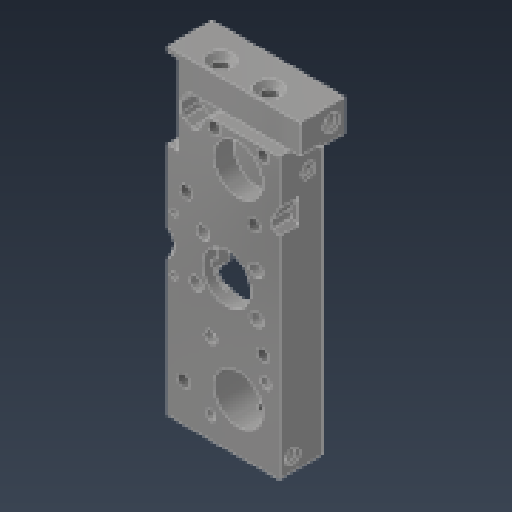
# Autodesk Inventor part: LeftGearbox
Saved by Autodesk Inventor 2027.1 (Build 311270010, 270A)
## iProperties
Created: 2026-04-13
Part Number: LeftGearbox
Material: Steel
Document SubType Name: Modeling
Designer: szymo
Density: 7.85 g/cm^3
Appearance: Nylon 6(1)
Mass: 68.9127 g
Surface Area: 68.8445 cm^2
Volume: 8.77869 cm^3
Author: szymo
Autodesk Inventor part; units mm, degrees
(part 1 of 2)
ref_plane "YZ Plane" through (0, 0, 0) normal (1, 0, 0) x (0, 1, 0)
ref_plane "XZ Plane" through (0, 0, 0) normal (0, 1, 0) x (-1, 0, 0)
ref_plane "XY Plane" through (0, 0, 0) normal (0, 0, 1) x (1, 0, 0)
sketch "Sketch1" plane through (0, 0, 0) normal (0, 0, 1) x (1, 0, 0)
  circle A0 centre (14.7, -55.637072) radius 14.7 construction
  circle A1 centre (14.7, -55.637072) radius 14 construction
  circle A2 centre (14.7, -55.637072) radius 5
  circle A3 centre (14.7, -14.7) radius 5
  circle A4 centre (14.7, -14.7) radius 14 construction
  circle A5 centre (14.7, -14.7) radius 14.7 construction
  circle A6 centre (12.35, -35.272213) radius 5
  circle A7 centre (9.001972, -47.419258) radius 8 construction
  circle A8 centre (9.001972, -47.419258) radius 4.2 construction
  circle A9 centre (12.35, -35.272213) radius 9.6 construction
  line L0 (23.1, -65.837072) -> (0, -65.837072)
  line L1 (0, -65.837072) -> (0, 0)
  line L2 (0, 0) -> (23.1, 0)
  line L3 (23.1, 0) -> (23.1, -65.837072)
  circle A10 centre (12.35, -35.272213) radius 10
  circle A11 centre (9.001972, -47.419258) radius 8.4
  line L4 (29.4, -55.637072) -> (23.1, -55.637072)
  line L5 (14.7, -55.637072) -> (23.1, -55.637072) construction
  line L6 (5.96251, -12.542159) -> (1.960875, -10.231814) construction
  arc A12 (4.460875, -5.901687) -> (1.960875, -10.231814) centre (14.7, -14.7) ccw construction
  line L7 (4.460875, -5.901687) -> (8.46251, -8.212032)
  arc A13 (8.46251, -8.212032) -> (5.96251, -12.542159) centre (14.7, -14.7) ccw construction
  arc A14 (24.939125, -23.498313) -> (27.439125, -19.168186) centre (14.7, -14.7) ccw
  line L8 (27.439125, -19.168186) -> (23.43749, -16.857841)
  arc A15 (20.93749, -21.187968) -> (23.43749, -16.857841) centre (14.7, -14.7) ccw construction
  line L9 (20.93749, -21.187968) -> (24.939125, -23.498313) construction
  line L10 (20.93749, -21.187968) -> (23.43749, -16.857841)
  line L11 (4.460875, -5.901687) -> (23.1, -5.901687)
  line L12 (5.96251, -12.542159) -> (23.1, -12.542159)
  line L13 (5.96251, -12.542159) -> (8.46251, -8.212032)
  line L14 (23.1, -6.5) -> (27.4, -6.5)
  line L15 (27.4, -6.5) -> (27.4, 0)
  line L16 (27.4, 0) -> (23.1, 0)
  circle A16 centre (9.001972, -47.419258) radius 4.6
  circle A17 centre (14.7, -55.637072) radius 14.7
  circle A18 centre (14.7, -55.637072) radius 14
  circle A19 centre (9.043146, -61.293926) radius 1.05643
  circle A20 centre (20.356854, -49.980218) radius 1.05643
  circle A21 centre (14.7, -55.637072) radius 5
  circle A22 centre (14.7, -55.637072) radius 14
  circle A23 centre (14.7, -14.7) radius 14.7
  circle A24 centre (14.7, -14.7) radius 14
  line L17 (6.887728, -8.457532) -> (4.702907, -7.196125)
  arc A25 (4.702907, -7.196125) -> (3.202907, -9.794201) centre (14.7, -14.7) ccw
  line L18 (3.202907, -9.794201) -> (5.387728, -11.055608)
  arc A26 (6.887728, -8.457532) -> (5.387728, -11.055608) centre (14.7, -14.7) ccw
  arc A27 (24.697093, -22.203875) -> (26.197093, -19.605799) centre (14.7, -14.7) ccw
  line L19 (26.197093, -19.605799) -> (24.012272, -18.344392)
  arc A28 (22.512272, -20.942468) -> (24.012272, -18.344392) centre (14.7, -14.7) ccw
  line L20 (22.512272, -20.942468) -> (24.697093, -22.203875)
  circle A29 centre (14.7, -14.7) radius 5
  circle A30 centre (14.7, -14.7) radius 14
  arc A31 (9.833797, -26.007834) -> (9.773924, -27.434717) centre (15.759046, -26.971155) ccw
  arc A32 (10.322105, -25.888842) -> (9.833797, -26.007834) centre (12.35, -35.272213) ccw
  arc A33 (11.031695, -27.128223) -> (10.322105, -25.888842) centre (5.50427, -29.470047) ccw
  arc A34 (11.459725, -27.070389) -> (11.031695, -27.128223) centre (12.35, -35.272213) ccw
  arc A35 (11.814954, -25.687134) -> (11.459725, -27.070389) centre (17.410437, -27.861334) ccw
  arc A36 (12.317332, -25.672268) -> (11.814954, -25.687134) centre (12.35, -35.272213) ccw
  arc A37 (12.753733, -27.032097) -> (12.317332, -25.672268) centre (6.860203, -28.173531) ccw
  arc A38 (13.184434, -27.06452) -> (12.753733, -27.032097) centre (12.35, -35.272213) ccw
  arc A39 (13.819496, -25.785349) -> (13.184434, -27.06452) centre (18.840663, -29.075403) ccw
  arc A40 (14.313986, -25.875258) -> (13.819496, -25.785349) centre (12.35, -35.272213) ccw
  arc A41 (14.458127, -27.296105) -> (14.313986, -25.875258) centre (8.456067, -27.187262) ccw
  arc A42 (14.872675, -27.417366) -> (14.458127, -27.296105) centre (12.35, -35.272213) ccw
  arc A43 (15.759814, -26.298185) -> (14.872675, -27.417366) centre (19.987215, -30.560303) ccw
  arc A44 (16.224805, -26.48894) -> (15.759814, -26.298185) centre (12.35, -35.272213) ccw
  arc A45 (16.070386, -27.908706) -> (16.224805, -26.48894) centre (10.222115, -26.554343) ccw
  arc A46 (16.450663, -28.113507) -> (16.070386, -27.908706) centre (12.35, -35.272213) ccw
  arc A47 (17.551107, -27.20323) -> (16.450663, -28.113507) centre (20.799985, -32.251136) ccw
  arc A48 (17.966277, -27.486493) -> (17.551107, -27.20323) centre (12.35, -35.272213) ccw
  arc A49 (17.520045, -28.843128) -> (17.966277, -27.486493) centre (12.081161, -26.302437) ccw
  arc A50 (17.849432, -29.122518) -> (17.520045, -28.843128) centre (12.35, -35.272213) ccw
  arc A51 (19.115086, -28.460927) -> (17.849432, -29.122518) centre (21.24345, -34.074005) ccw
  arc A52 (19.46229, -28.824319) -> (19.115086, -28.460927) centre (12.35, -35.272213) ccw
  arc A53 (18.743749, -30.058532) -> (19.46229, -28.824319) centre (13.951957, -26.442554) ccw
  arc A54 (19.00785, -30.4003) -> (18.743749, -30.058532) centre (12.35, -35.272213) ccw
  arc A55 (20.383398, -30.01631) -> (19.00785, -30.4003) centre (21.298228, -35.94924) ccw
  arc A56 (20.647462, -30.443949) -> (20.383398, -30.01631) centre (12.35, -35.272213) ccw
  arc A57 (19.688016, -31.501799) -> (20.647462, -30.443949) centre (15.75274, -26.968568) ccw
  arc A58 (19.875288, -31.891008) -> (19.688016, -31.501799) centre (12.35, -35.272213) ccw
  arc A59 (21.300613, -31.801402) -> (19.875288, -31.891008) centre (20.961926, -37.794887) ccw
  arc A60 (21.469995, -32.274598) -> (21.300613, -31.801402) centre (12.35, -35.272213) ccw
  arc A61 (20.311576, -33.10985) -> (21.469995, -32.274598) centre (17.404807, -27.857492) ccw
  arc A62 (20.413834, -33.529491) -> (20.311576, -33.10985) centre (12.35, -35.272213) ccw
  arc A63 (21.826643, -33.738185) -> (20.413834, -33.529491) centre (20.249241, -39.53028) ccw
  arc A64 (21.89394, -34.236256) -> (21.826643, -33.738185) centre (12.35, -35.272213) ccw
  arc A65 (20.587177, -34.812408) -> (21.89394, -34.236256) centre (18.835954, -29.070475) ccw
  arc A66 (20.599952, -35.244139) -> (20.587177, -34.812408) centre (12.35, -35.272213) ccw
  arc A67 (21.938498, -35.742012) -> (20.599952, -35.244139) centre (19.191321, -41.079576) ccw
  arc A68 (21.90077, -36.243191) -> (21.938498, -35.742012) centre (12.35, -35.272213) ccw
  arc A69 (20.502773, -36.535061) -> (21.90077, -36.243191) centre (19.983634, -30.554504) ccw
  arc A70 (20.425508, -36.960014) -> (20.502773, -36.535061) centre (12.35, -35.272213) ccw
  arc A71 (21.631289, -37.725306) -> (20.425508, -36.960014) centre (17.834403, -42.375062) ccw
  arc A72 (21.490185, -38.207689) -> (21.631289, -37.725306) centre (12.35, -35.272213) ccw
  arc A73 (20.062055, -38.202522) -> (21.490185, -38.207689) centre (20.797688, -32.244719) ccw
  arc A74 (19.898125, -38.602124) -> (20.062055, -38.202522) centre (12.35, -35.272213) ccw
  arc A75 (20.918444, -39.601389) -> (19.898125, -38.602124) centre (16.237791, -43.360119) ccw
  arc A76 (20.68013, -40.043893) -> (20.918444, -39.601389) centre (12.35, -35.272213) ccw
  arc A77 (19.284282, -39.741914) -> (20.68013, -40.043893) centre (21.242537, -34.06725) ccw
  arc A78 (19.040853, -40.0987) -> (19.284282, -39.741914) centre (12.35, -35.272213) ccw
  arc A79 (19.831117, -41.288266) -> (19.040853, -40.0987) centre (14.471263, -43.991696) ccw
  arc A80 (19.506008, -41.671552) -> (19.831117, -41.288266) centre (12.35, -35.272213) ccw
  arc A81 (18.203449, -41.085958) -> (19.506008, -41.671552) centre (21.298739, -35.942444) ccw
  arc A82 (17.891159, -41.384337) -> (18.203449, -41.085958) centre (12.35, -35.272213) ccw
  arc A83 (18.416829, -42.712212) -> (17.891159, -41.384337) centre (12.612026, -44.24219) ccw
  arc A84 (18.019135, -43.019529) -> (18.416829, -42.712212) centre (12.35, -35.272213) ccw
  arc A85 (16.866791, -42.175915) -> (18.019135, -43.019529) centre (20.963839, -37.788345) ccw
  arc A86 (16.499289, -42.402844) -> (16.866791, -42.175915) centre (12.35, -35.272213) ccw
  arc A87 (16.737391, -43.810995) -> (16.499289, -42.402844) centre (10.741337, -44.100653) ccw
  arc A88 (16.284493, -44.028911) -> (16.737391, -43.810995) centre (12.35, -35.272213) ccw
  arc A89 (15.332728, -42.964146) -> (16.284493, -44.028911) centre (20.252473, -39.524279) ccw
  arc A90 (14.926076, -43.109708) -> (15.332728, -42.964146) centre (12.35, -35.272213) ccw
  arc A91 (14.866203, -44.536592) -> (14.926076, -43.109708) centre (8.940954, -43.57327) ccw
  arc A92 (14.377895, -44.655583) -> (14.866203, -44.536592) centre (12.35, -35.272213) ccw
  arc A93 (13.668305, -43.416203) -> (14.377895, -44.655583) centre (19.19573, -41.074378) ccw
  arc A94 (13.240275, -43.474036) -> (13.668305, -43.416203) centre (12.35, -35.272213) ccw
  arc A95 (12.885046, -44.857291) -> (13.240275, -43.474036) centre (7.289563, -42.683091) ccw
  arc A96 (12.382668, -44.872157) -> (12.885046, -44.857291) centre (12.35, -35.272213) ccw
  arc A97 (11.946267, -43.512328) -> (12.382668, -44.872157) centre (17.839797, -42.370894) ccw
  arc A98 (11.515566, -43.479905) -> (11.946267, -43.512328) centre (12.35, -35.272213) ccw
  arc A99 (10.880504, -44.759076) -> (11.515566, -43.479905) centre (5.859337, -41.469022) ccw
  arc A100 (10.386014, -44.669167) -> (10.880504, -44.759076) centre (12.35, -35.272213) ccw
  arc A101 (10.241873, -43.248321) -> (10.386014, -44.669167) centre (16.243933, -43.357164) ccw
  arc A102 (9.827325, -43.127059) -> (10.241873, -43.248321) centre (12.35, -35.272213) ccw
  arc A103 (8.940186, -44.24624) -> (9.827325, -43.127059) centre (4.712785, -39.984122) ccw
  arc A104 (8.475195, -44.055486) -> (8.940186, -44.24624) centre (12.35, -35.272213) ccw
  arc A105 (8.629614, -42.635719) -> (8.475195, -44.055486) centre (14.477885, -43.990082) ccw
  arc A106 (8.249337, -42.430918) -> (8.629614, -42.635719) centre (12.35, -35.272213) ccw
  arc A107 (7.148893, -43.341196) -> (8.249337, -42.430918) centre (3.900015, -38.293289) ccw
  arc A108 (6.733723, -43.057933) -> (7.148893, -43.341196) centre (12.35, -35.272213) ccw
  arc A109 (7.179955, -41.701297) -> (6.733723, -43.057933) centre (12.618839, -44.241988) ccw
  arc A110 (6.850568, -41.421907) -> (7.179955, -41.701297) centre (12.35, -35.272213) ccw
  arc A111 (5.584914, -42.083498) -> (6.850568, -41.421907) centre (3.45655, -36.470421) ccw
  arc A112 (5.23771, -41.720106) -> (5.584914, -42.083498) centre (12.35, -35.272213) ccw
  arc A113 (5.956251, -40.485894) -> (5.23771, -41.720106) centre (10.748043, -44.101872) ccw
  arc A114 (5.69215, -40.144125) -> (5.956251, -40.485894) centre (12.35, -35.272213) ccw
  arc A115 (4.316602, -40.528115) -> (5.69215, -40.144125) centre (3.401772, -34.595185) ccw
  arc A116 (4.052538, -40.100476) -> (4.316602, -40.528115) centre (12.35, -35.272213) ccw
  arc A117 (5.011984, -39.042627) -> (4.052538, -40.100476) centre (8.94726, -43.575857) ccw
  arc A118 (4.824712, -38.653418) -> (5.011984, -39.042627) centre (12.35, -35.272213) ccw
  arc A119 (3.399387, -38.743023) -> (4.824712, -38.653418) centre (3.738074, -32.749539) ccw
  arc A120 (3.230005, -38.269828) -> (3.399387, -38.743023) centre (12.35, -35.272213) ccw
  arc A121 (4.388424, -37.434575) -> (3.230005, -38.269828) centre (7.295193, -42.686933) ccw
  arc A122 (4.286166, -37.014935) -> (4.388424, -37.434575) centre (12.35, -35.272213) ccw
  arc A123 (2.873357, -36.806241) -> (4.286166, -37.014935) centre (4.450759, -31.014145) ccw
  arc A124 (2.80606, -36.308169) -> (2.873357, -36.806241) centre (12.35, -35.272213) ccw
  arc A125 (4.112823, -35.732018) -> (2.80606, -36.308169) centre (5.864046, -41.47395) ccw
  arc A126 (4.100048, -35.300287) -> (4.112823, -35.732018) centre (12.35, -35.272213) ccw
  arc A127 (2.761502, -34.802414) -> (4.100048, -35.300287) centre (5.508679, -29.464849) ccw
  arc A128 (2.79923, -34.301234) -> (2.761502, -34.802414) centre (12.35, -35.272213) ccw
  arc A129 (4.197227, -34.009364) -> (2.79923, -34.301234) centre (4.716366, -39.989922) ccw
  arc A130 (4.274492, -33.584412) -> (4.197227, -34.009364) centre (12.35, -35.272213) ccw
  arc A131 (3.068711, -32.819119) -> (4.274492, -33.584412) centre (6.865597, -28.169364) ccw
  arc A132 (3.209815, -32.336736) -> (3.068711, -32.819119) centre (12.35, -35.272213) ccw
  arc A133 (4.637945, -32.341904) -> (3.209815, -32.336736) centre (3.902312, -38.299707) ccw
  arc A134 (4.801875, -31.942302) -> (4.637945, -32.341904) centre (12.35, -35.272213) ccw
  arc A135 (3.781556, -30.943037) -> (4.801875, -31.942302) centre (8.462209, -27.184306) ccw
  arc A136 (4.01987, -30.500532) -> (3.781556, -30.943037) centre (12.35, -35.272213) ccw
  arc A137 (5.415718, -30.802512) -> (4.01987, -30.500532) centre (3.457463, -36.477176) ccw
  arc A138 (5.659147, -30.445725) -> (5.415718, -30.802512) centre (12.35, -35.272213) ccw
  arc A139 (4.868883, -29.25616) -> (5.659147, -30.445725) centre (10.228737, -26.552729) ccw
  arc A140 (5.193992, -28.872873) -> (4.868883, -29.25616) centre (12.35, -35.272213) ccw
  arc A141 (6.496551, -29.458467) -> (5.193992, -28.872873) centre (3.401261, -34.601982) ccw
  arc A142 (6.808841, -29.160089) -> (6.496551, -29.458467) centre (12.35, -35.272213) ccw
  arc A143 (6.283171, -27.832213) -> (6.808841, -29.160089) centre (12.087974, -26.302236) ccw
  arc A144 (6.680865, -27.524896) -> (6.283171, -27.832213) centre (12.35, -35.272213) ccw
  arc A145 (7.833209, -28.368511) -> (6.680865, -27.524896) centre (3.736161, -32.75608) ccw
  arc A146 (8.200711, -28.141582) -> (7.833209, -28.368511) centre (12.35, -35.272213) ccw
  arc A147 (7.962609, -26.733431) -> (8.200711, -28.141582) centre (13.958663, -26.443773) ccw
  arc A148 (8.415507, -26.515514) -> (7.962609, -26.733431) centre (12.35, -35.272213) ccw
  arc A149 (9.367272, -27.58028) -> (8.415507, -26.515514) centre (4.447527, -31.020146) ccw
  arc A150 (9.773924, -27.434717) -> (9.367272, -27.58028) centre (12.35, -35.272213) ccw
  circle A151 centre (9.001972, -47.419258) radius 1.25
  arc A152 (9.305411, -54.287558) -> (9.772861, -55.382029) centre (14.106978, -52.883865) ccw
  arc A153 (8.945536, -54.294026) -> (9.305411, -54.287558) centre (9.001972, -47.419258) ccw
  arc A154 (8.517718, -55.404588) -> (8.945536, -54.294026) centre (4.09663, -53.063781) ccw
  arc A155 (8.100462, -55.368301) -> (8.517718, -55.404588) centre (9.001972, -47.419258) ccw
  arc A156 (7.870781, -54.200558) -> (8.100462, -55.368301) centre (12.859266, -53.825841) ccw
  arc A157 (7.517425, -54.132063) -> (7.870781, -54.200558) centre (9.001972, -47.419258) ccw
  arc A158 (6.868057, -55.129407) -> (7.517425, -54.132063) centre (3.030261, -51.920557) ccw
  arc A159 (6.467463, -55.007161) -> (6.868057, -55.129407) centre (9.001972, -47.419258) ccw
  arc A160 (6.485588, -53.817182) -> (6.467463, -55.007161) centre (11.442971, -54.487818) ccw
  arc A161 (6.154195, -53.676717) -> (6.485588, -53.817182) centre (9.001972, -47.419258) ccw
  arc A162 (5.311658, -54.517256) -> (6.154195, -53.676717) centre (2.224885, -50.580604) ccw
  arc A163 (4.945234, -54.314393) -> (5.311658, -54.517256) centre (9.001972, -47.419258) ccw
  arc A164 (5.210374, -53.154187) -> (4.945234, -54.314393) centre (9.919993, -54.840865) ccw
  arc A165 (4.915427, -52.947891) -> (5.210374, -53.154187) centre (9.001972, -47.419258) ccw
  arc A166 (3.916543, -53.594889) -> (4.915427, -52.947891) centre (1.715699, -49.102486) ccw
  arc A167 (3.600305, -53.320274) -> (3.916543, -53.594889) centre (9.001972, -47.419258) ccw
  arc A168 (4.100871, -52.240548) -> (3.600305, -53.320274) centre (8.356893, -54.869553) ccw
  arc A169 (3.855261, -51.977436) -> (4.100871, -52.240548) centre (9.001972, -47.419258) ccw
  arc A170 (2.743686, -52.402616) -> (3.855261, -51.977436) centre (1.524959, -47.550802) ccw
  arc A171 (2.491454, -52.068253) -> (2.743686, -52.402616) centre (9.001972, -47.419258) ccw
  arc A172 (3.205569, -51.116195) -> (2.491454, -52.068253) centre (6.821986, -54.572627) ccw
  arc A173 (3.02003, -50.807768) -> (3.205569, -51.116195) centre (9.001972, -47.419258) ccw
  arc A174 (1.844346, -50.992547) -> (3.02003, -50.807768) centre (1.661, -45.993369) ccw
  arc A175 (1.667144, -50.613049) -> (1.844346, -50.992547) centre (9.001972, -47.419258) ccw
  arc A176 (2.563598, -49.830268) -> (1.667144, -50.613049) centre (5.382355, -53.963064) ccw
  arc A177 (2.446239, -49.490005) -> (2.563598, -49.830268) centre (9.001972, -47.419258) ccw
  arc A178 (1.257829, -49.426308) -> (2.446239, -49.490005) centre (2.117877, -44.498254) ccw
  arc A179 (1.163401, -49.01826) -> (1.257829, -49.426308) centre (9.001972, -47.419258) ccw
  arc A180 (2.203015, -48.438968) -> (1.163401, -49.01826) centre (4.100919, -53.067505) ccw
  arc A181 (2.158965, -48.081741) -> (2.203015, -48.438968) centre (9.001972, -47.419258) ccw
  arc A182 (1.009768, -47.772351) -> (2.158965, -48.081741) centre (2.875622, -43.130802) ccw
  arc A183 (1.002241, -47.353588) -> (1.009768, -47.772351) centre (9.001972, -47.419258) ccw
  arc A184 (2.139578, -47.003102) -> (1.002241, -47.353588) centre (3.033682, -51.925091) ccw
  arc A185 (2.170763, -46.644523) -> (2.139578, -47.003102) centre (9.001972, -47.419258) ccw
  arc A186 (1.111004, -46.102963) -> (2.170763, -46.644523) centre (3.901117, -41.950775) ccw
  arc A187 (1.190708, -45.691785) -> (1.111004, -46.102963) centre (9.001972, -47.419258) ccw
  arc A188 (2.376062, -45.585425) -> (1.190708, -45.691785) centre (2.227288, -50.585751) ccw
  arc A189 (2.481118, -45.241165) -> (2.376062, -45.585425) centre (9.001972, -47.419258) ccw
  arc A190 (1.557114, -44.491103) -> (2.481118, -45.241165) centre (5.149545, -41.009747) ccw
  arc A191 (1.720565, -44.105482) -> (1.557114, -44.491103) centre (9.001972, -47.419258) ccw
  arc A192 (2.902129, -44.247894) -> (1.720565, -44.105482) centre (1.71698, -49.10802) ccw
  arc A193 (3.076465, -43.932999) -> (2.902129, -44.247894) centre (9.001972, -47.419258) ccw
  arc A194 (2.328599, -43.007217) -> (3.076465, -43.932999) centre (6.566342, -40.348846) ccw
  arc A195 (2.568654, -42.664006) -> (2.328599, -43.007217) centre (9.001972, -47.419258) ccw
  arc A196 (3.694789, -43.048968) -> (2.568654, -42.664006) centre (1.525061, -47.556481) ccw
  arc A197 (3.930785, -42.7772) -> (3.694789, -43.048968) centre (9.001972, -47.419258) ccw
  arc A198 (3.391744, -41.716159) -> (3.930785, -42.7772) centre (8.089587, -39.996955) ccw
  arc A199 (3.697909, -41.430358) -> (3.391744, -41.716159) centre (9.001972, -47.419258) ccw
  arc A200 (4.719398, -42.041044) -> (3.697909, -41.430358) centre (1.659919, -45.998945) ccw
  arc A201 (5.006741, -41.824282) -> (4.719398, -42.041044) centre (9.001972, -47.419258) ccw
  arc A202 (4.700082, -40.674353) -> (5.006741, -41.824282) centre (9.652709, -39.969455) ccw
  arc A203 (5.058978, -40.458453) -> (4.700082, -40.674353) centre (9.001972, -47.419258) ccw
  arc A204 (5.931176, -41.268173) -> (5.058978, -40.458453) centre (2.11566, -44.503484) ccw
  arc A205 (6.257307, -41.11589) -> (5.931176, -41.268173) centre (9.001972, -47.419258) ccw
  arc A206 (6.196433, -39.927332) -> (6.257307, -41.11589) centre (11.18739, -40.267547) ccw
  arc A207 (6.592375, -39.790769) -> (6.196433, -39.927332) centre (9.001972, -47.419258) ccw
  arc A208 (7.277163, -40.764135) -> (6.592375, -39.790769) centre (2.872366, -43.135456) ccw
  arc A209 (7.627829, -40.682986) -> (7.277163, -40.764135) centre (9.001972, -47.419258) ccw
  arc A210 (7.815399, -39.507744) -> (7.627829, -40.682986) centre (12.626557, -40.878203) ccw
  arc A211 (8.231082, -39.456486) -> (7.815399, -39.507744) centre (9.001972, -47.419258) ccw
  arc A212 (8.698532, -40.550958) -> (8.231082, -39.456486) centre (3.896965, -41.954651) ccw
  arc A213 (9.058407, -40.544489) -> (8.698532, -40.550958) centre (9.001972, -47.419258) ccw
  arc A214 (9.486225, -39.433928) -> (9.058407, -40.544489) centre (13.907313, -41.774735) ccw
  arc A215 (9.903481, -39.470215) -> (9.486225, -39.433928) centre (9.001972, -47.419258) ccw
  arc A216 (10.133163, -40.637958) -> (9.903481, -39.470215) centre (5.144678, -41.012675) ccw
  arc A217 (10.486518, -40.706453) -> (10.133163, -40.637958) centre (9.001972, -47.419258) ccw
  arc A218 (11.135886, -39.709108) -> (10.486518, -40.706453) centre (14.973682, -42.917959) ccw
  arc A219 (11.53648, -39.831355) -> (11.135886, -39.709108) centre (9.001972, -47.419258) ccw
  arc A220 (11.518355, -41.021333) -> (11.53648, -39.831355) centre (6.560972, -40.350698) ccw
  arc A221 (11.849748, -41.161799) -> (11.518355, -41.021333) centre (9.001972, -47.419258) ccw
  arc A222 (12.692286, -40.321259) -> (11.849748, -41.161799) centre (15.779059, -44.257911) ccw
  arc A223 (13.058709, -40.524123) -> (12.692286, -40.321259) centre (9.001972, -47.419258) ccw
  arc A224 (12.793569, -41.684329) -> (13.058709, -40.524123) centre (8.08395, -39.997651) ccw
  arc A225 (13.088516, -41.890625) -> (12.793569, -41.684329) centre (9.001972, -47.419258) ccw
  arc A226 (14.0874, -41.243627) -> (13.088516, -41.890625) centre (16.288244, -45.73603) ccw
  arc A227 (14.403638, -41.518241) -> (14.0874, -41.243627) centre (9.001972, -47.419258) ccw
  arc A228 (13.903073, -42.597968) -> (14.403638, -41.518241) centre (9.64705, -39.968963) ccw
  arc A229 (14.148683, -42.861079) -> (13.903073, -42.597968) centre (9.001972, -47.419258) ccw
  arc A230 (15.260257, -42.4359) -> (14.148683, -42.861079) centre (16.478984, -47.287714) ccw
  arc A231 (15.512489, -42.770262) -> (15.260257, -42.4359) centre (9.001972, -47.419258) ccw
  arc A232 (14.798374, -43.722321) -> (15.512489, -42.770262) centre (11.181957, -40.265889) ccw
  arc A233 (14.983913, -44.030748) -> (14.798374, -43.722321) centre (9.001972, -47.419258) ccw
  arc A234 (16.159597, -43.845969) -> (14.983913, -44.030748) centre (16.342943, -48.845147) ccw
  arc A235 (16.336799, -44.225467) -> (16.159597, -43.845969) centre (9.001972, -47.419258) ccw
  arc A236 (15.440345, -45.008248) -> (16.336799, -44.225467) centre (12.621588, -40.875452) ccw
  arc A237 (15.557704, -45.348511) -> (15.440345, -45.008248) centre (9.001972, -47.419258) ccw
  arc A238 (16.746114, -45.412208) -> (15.557704, -45.348511) centre (15.886066, -50.340261) ccw
  arc A239 (16.840542, -45.820255) -> (16.746114, -45.412208) centre (9.001972, -47.419258) ccw
  arc A240 (15.800929, -46.399547) -> (16.840542, -45.820255) centre (13.903024, -41.77101) ccw
  arc A241 (15.844978, -46.756775) -> (15.800929, -46.399547) centre (9.001972, -47.419258) ccw
  arc A242 (16.994176, -47.066164) -> (15.844978, -46.756775) centre (15.128321, -51.707714) ccw
  arc A243 (17.001702, -47.484928) -> (16.994176, -47.066164) centre (9.001972, -47.419258) ccw
  arc A244 (15.864365, -47.835413) -> (17.001702, -47.484928) centre (14.970261, -42.913424) ccw
  arc A245 (15.83318, -48.193993) -> (15.864365, -47.835413) centre (9.001972, -47.419258) ccw
  arc A246 (16.892939, -48.735553) -> (15.83318, -48.193993) centre (14.102826, -52.887741) ccw
  arc A247 (16.813235, -49.14673) -> (16.892939, -48.735553) centre (9.001972, -47.419258) ccw
  arc A248 (15.627881, -49.253091) -> (16.813235, -49.14673) centre (15.776655, -44.252765) ccw
  arc A249 (15.522825, -49.597351) -> (15.627881, -49.253091) centre (9.001972, -47.419258) ccw
  arc A250 (16.446829, -50.347413) -> (15.522825, -49.597351) centre (12.854398, -53.828769) ccw
  arc A251 (16.283379, -50.733034) -> (16.446829, -50.347413) centre (9.001972, -47.419258) ccw
  arc A252 (15.101814, -50.590621) -> (16.283379, -50.733034) centre (16.286963, -45.730496) ccw
  arc A253 (14.927478, -50.905516) -> (15.101814, -50.590621) centre (9.001972, -47.419258) ccw
  arc A254 (15.675344, -51.831299) -> (14.927478, -50.905516) centre (11.437601, -54.48967) ccw
  arc A255 (15.43529, -52.17451) -> (15.675344, -51.831299) centre (9.001972, -47.419258) ccw
  arc A256 (14.309154, -51.789548) -> (15.43529, -52.17451) centre (16.478882, -47.282035) ccw
  arc A257 (14.073158, -52.061315) -> (14.309154, -51.789548) centre (9.001972, -47.419258) ccw
  arc A258 (14.6122, -53.122357) -> (14.073158, -52.061315) centre (9.914356, -54.84156) ccw
  arc A259 (14.306034, -53.408158) -> (14.6122, -53.122357) centre (9.001972, -47.419258) ccw
  arc A260 (13.284545, -52.797472) -> (14.306034, -53.408158) centre (16.344024, -48.83957) ccw
  arc A261 (12.997202, -53.014234) -> (13.284545, -52.797472) centre (9.001972, -47.419258) ccw
  arc A262 (13.303862, -54.164163) -> (12.997202, -53.014234) centre (8.351234, -54.869061) ccw
  arc A263 (12.944965, -54.380063) -> (13.303862, -54.164163) centre (9.001972, -47.419258) ccw
  arc A264 (12.072767, -53.570342) -> (12.944965, -54.380063) centre (15.888283, -50.335032) ccw
  arc A265 (11.746636, -53.722625) -> (12.072767, -53.570342) centre (9.001972, -47.419258) ccw
  arc A266 (11.80751, -54.911184) -> (11.746636, -53.722625) centre (6.816554, -54.570969) ccw
  arc A267 (11.411568, -55.047747) -> (11.80751, -54.911184) centre (9.001972, -47.419258) ccw
  arc A268 (10.72678, -54.074381) -> (11.411568, -55.047747) centre (15.131577, -51.70306) ccw
  arc A269 (10.376114, -54.15553) -> (10.72678, -54.074381) centre (9.001972, -47.419258) ccw
  arc A270 (10.188544, -55.330771) -> (10.376114, -54.15553) centre (5.377386, -53.960313) ccw
  arc A271 (9.772861, -55.382029) -> (10.188544, -55.330771) centre (9.001972, -47.419258) ccw
  circle A272 centre (9.001972, -47.419258) radius 1.25
  arc A273 (10.079754, -44.780909) -> (10.069196, -43.357112) centre (6.439072, -44.095967) ccw
  arc A274 (10.414907, -44.944159) -> (10.079754, -44.780909) centre (9.001972, -47.419258) ccw
  arc A275 (11.542475, -44.074734) -> (10.414907, -44.944159) centre (13.198609, -47.388482) ccw
  arc A276 (11.957289, -44.434949) -> (11.542475, -44.074734) centre (9.001972, -47.419258) ccw
  arc A277 (11.254533, -45.673272) -> (11.957289, -44.434949) centre (8.444081, -43.259754) ccw
  arc A278 (11.463159, -45.982227) -> (11.254533, -45.673272) centre (9.001972, -47.419258) ccw
  arc A279 (12.874374, -45.793066) -> (11.463159, -45.982227) centre (12.651754, -49.490924) ccw
  arc A280 (13.053506, -46.312429) -> (12.874374, -45.793066) centre (9.001972, -47.419258) ccw
  arc A281 (11.82574, -47.03347) -> (13.053506, -46.312429) centre (10.598576, -43.538077) ccw
  arc A282 (11.851938, -47.405347) -> (11.82574, -47.03347) centre (9.001972, -47.419258) ccw
  arc A283 (13.168666, -47.947136) -> (11.851938, -47.405347) centre (11.126943, -51.038265) ccw
  arc A284 (13.064118, -48.486483) -> (13.168666, -47.947136) centre (9.001972, -47.419258) ccw
  arc A285 (11.64032, -48.49704) -> (13.064118, -48.486483) centre (12.325262, -44.856358) ccw
  arc A286 (11.47707, -48.832193) -> (11.64032, -48.49704) centre (9.001972, -47.419258) ccw
  arc A287 (12.346496, -49.959761) -> (11.47707, -48.832193) centre (9.032747, -51.615895) ccw
  arc A288 (11.986281, -50.374575) -> (12.346496, -49.959761) centre (9.001972, -47.419258) ccw
  arc A289 (10.747957, -49.671819) -> (11.986281, -50.374575) centre (13.161475, -46.861367) ccw
  arc A290 (10.439002, -49.880445) -> (10.747957, -49.671819) centre (9.001972, -47.419258) ccw
  arc A291 (10.628163, -51.29166) -> (10.439002, -49.880445) centre (6.930305, -51.06904) ccw
  arc A292 (10.108801, -51.470792) -> (10.628163, -51.29166) centre (9.001972, -47.419258) ccw
  arc A293 (9.387759, -50.243026) -> (10.108801, -51.470792) centre (12.883153, -49.015862) ccw
  arc A294 (9.015883, -50.269224) -> (9.387759, -50.243026) centre (9.001972, -47.419258) ccw
  arc A295 (8.474093, -51.585953) -> (9.015883, -50.269224) centre (5.382965, -49.544229) ccw
  arc A296 (7.934747, -51.481404) -> (8.474093, -51.585953) centre (9.001972, -47.419258) ccw
  arc A297 (7.924189, -50.057607) -> (7.934747, -51.481404) centre (11.564871, -50.742548) ccw
  arc A298 (7.589036, -49.894356) -> (7.924189, -50.057607) centre (9.001972, -47.419258) ccw
  arc A299 (6.461468, -50.763782) -> (7.589036, -49.894356) centre (4.805334, -47.450034) ccw
  arc A300 (6.046655, -50.403567) -> (6.461468, -50.763782) centre (9.001972, -47.419258) ccw
  arc A301 (6.74941, -49.165244) -> (6.046655, -50.403567) centre (9.559862, -51.578762) ccw
  arc A302 (6.540784, -48.856288) -> (6.74941, -49.165244) centre (9.001972, -47.419258) ccw
  arc A303 (5.129569, -49.045449) -> (6.540784, -48.856288) centre (5.352189, -45.347592) ccw
  arc A304 (4.950437, -48.526087) -> (5.129569, -49.045449) centre (9.001972, -47.419258) ccw
  arc A305 (6.178203, -47.805045) -> (4.950437, -48.526087) centre (7.405367, -51.300439) ccw
  arc A306 (6.152006, -47.433169) -> (6.178203, -47.805045) centre (9.001972, -47.419258) ccw
  arc A307 (4.835277, -46.89138) -> (6.152006, -47.433169) centre (6.877, -43.800251) ccw
  arc A308 (4.939825, -46.352033) -> (4.835277, -46.89138) centre (9.001972, -47.419258) ccw
  arc A309 (6.363623, -46.341475) -> (4.939825, -46.352033) centre (5.678681, -49.982157) ccw
  arc A310 (6.526873, -46.006322) -> (6.363623, -46.341475) centre (9.001972, -47.419258) ccw
  arc A311 (5.657447, -44.878755) -> (6.526873, -46.006322) centre (8.971196, -43.22262) ccw
  arc A312 (6.017662, -44.463941) -> (5.657447, -44.878755) centre (9.001972, -47.419258) ccw
  arc A313 (7.255986, -45.166696) -> (6.017662, -44.463941) centre (4.842468, -47.977149) ccw
  arc A314 (7.564941, -44.95807) -> (7.255986, -45.166696) centre (9.001972, -47.419258) ccw
  arc A315 (7.37578, -43.546855) -> (7.564941, -44.95807) centre (11.073638, -43.769475) ccw
  arc A316 (7.895142, -43.367724) -> (7.37578, -43.546855) centre (9.001972, -47.419258) ccw
  arc A317 (8.616184, -44.595489) -> (7.895142, -43.367724) centre (5.12079, -45.822654) ccw
  arc A318 (8.98806, -44.569292) -> (8.616184, -44.595489) centre (9.001972, -47.419258) ccw
  arc A319 (9.52985, -43.252563) -> (8.98806, -44.569292) centre (12.620978, -45.294287) ccw
  arc A320 (10.069196, -43.357112) -> (9.52985, -43.252563) centre (9.001972, -47.419258) ccw
  circle A321 centre (12.35, -35.272213) radius 4.8 construction
  line L21 (2.5, -1) -> (1, -1)
  line L22 (1, -1) -> (1, -17.5)
  line L23 (1, -17.5) -> (2.5, -17.5)
  line L24 (2.5, -17.5) -> (2.5, -1)
  line L25 (1.5, -1) -> (1.5, -17)
  line L26 (2.5, -1) -> (1.5, -1)
  line L27 (2.5, -17) -> (2.5, -1)
  line L28 (2.5, -17) -> (1.5, -17)
  line L29 (1, -17.5) -> (0, -17.5)
  line L30 (1, -1) -> (0, -1)
  point P0 (0, 0)
  point P1 (23.1, -8.689592)
  point P2 (3.954426, -40.704923)
  point P3 (16.776696, -44.239061)
  point P4 (13.27321, -40.186242)
  point P5 (9.039559, -39.019342)
  point P6 (13.056865, -45.247199)
  point P7 (6.63248, -43.476478)
  point P8 (16.595654, -51.010357)
  point P9 (9.70234, -55.79001)
  point P10 (0.26913, -17.5)
  point P11 (0, -14.7)
  point P12 (1, -1)
  point P13 (9.359596, -39.026874)
  point P14 (12.994507, -40.028746)
  dimension "d0" = 4.5
  dimension "d2" = 0.4
  dimension "d3" = 0.4
  dimension "d5" = 6.3
  dimension "d8" = 2
  dimension "d10" = 0.4
  dimension "d19" = 10
  dimension "d20" = 1
  dimension "d21" = 1
  dimension "d22" = 1
  dimension "d24" = 1
  dimension "d25" = 1
  dimension "d26" = 1
  dimension "d27" = 1
  dimension "d28" = 1
  dimension "d56" = 0.5
  dimension "d57" = 0.5
  dimension "d77" = 0
  dimension "d78" = 0
  dimension "d156" = 6.5
  constraints: 46 end point, 13 centre point, 11 point on line, 10 coincident, 9 perpendicular, 8 point on circle, 5 parallel, 5 tangent, 2 collinear, 2 horizontal, 2 horizontal alignment, 17 other
  measures "d5" distance of L4.start L4.end
  measures "d8" distance edge to line of A5 L15
  measures "d19" diameter of A6
  measures "d20" distance between parallel lines of L7 L17
  measures "d21" radial gap between concentric circles of A12 A25
  measures "d22" radial gap between concentric circles of A13 A26
  measures "d24" distance between parallel lines of L6 L18
  measures "d25" distance between parallel lines of L9 L20
  measures "d26" distance between parallel lines of L8 L19
  measures "d27" radial gap between concentric circles of A28 A15
  measures "d28" radial gap between concentric circles of A14 A27
  measures "d56" distance between parallel lines of L22 L25
  measures "d57" distance between parallel lines of L23 L28
  measures "d77" distance between parallel lines of L26 L30
  measures "d78" distance between parallel lines of L23 L29
  measures "d156" distance between parallel lines of L14 L16
extrude "Extrusion1" add sketch "Sketch1" against normal blind 1.6 contours A2 A11 A10 A18 L3 L0 | A2 A253 A252 A251 A250 A249 A248 A247 A246 A245 A244 A243 A242 A241 A240 A239 A238 A237 A236 A10 A11 | A11 A18 A178 A177 A176 A175 A174 A173 A172 A171 A170 A169 A168 A167 A166 A165 A164 A163 A162 A161 A160 A159 A158 A157 A156 A155 A154 A153 A152 A2 | A2 A152 A153 A154 A155 A156 A157 A158 A159 A160 A161 A162 A163 A164 A165 A166 A167 A168 A169 A170 A171 A172 A173 A174 A175 A176 A177 A178 A18 A16 A10 A236 A237 A238 A239 A240 A241 A242 A243 A244 A245 A246 A247 A248 A249 A250 A251 A252 A253 | A18 L0 A17 A11 | A11 A17 A178 A18 | A11 A88 A87 A86 A85 A84 A83 A18 A10 | A10 A236 A235 A89 A88 A11 | A17 L1 L29 A23 A10 A11 | A11 A10 A201 A200 A199 A198 A197 A196 A195 A194 A193 A192 A191 A190 A189 A188 A187 A186 A185 A184 A183 A182 A17 A180 A179 A178 | A178 A17 A180 A181 A182 A10 A16 A18 | A10 A16 A96 A95 A94 A93 A92 A91 A233 A234 A89 A235 A236 | A18 A83 A82 A17 A10 | A10 A17 L3 A18 | A88 A89 A235 A234 A232 A231 A230 A229 A228 A18 A11 | A11 A18 A83 A84 A85 A86 A87 A88 | A11 A116 A115 A114 A113 A204 A203 A202 A201 A10 | A10 A23 A147 A146 A145 A144 A143 A142 A141 A140 A139 A138 A137 A136 A135 A134 A133 A132 A131 A130 A129 A128 A127 A126 A125 A124 A123 A122 A121 A120 A119 A118 A117 A116 A11 | A178 A179 A180 A17 | A17 L0 L1 | A18 A311 A310 A309 A308 A307 A306 A305 A304 A303 A302 A301 A300 A299 A298 A297 A296 A295 A294 A293 A292 A291 A290 A289 A288 A287 A286 A285 A284 A283 A282 A281 A280 A279 A278 A277 A10 A16 | A16 A10 A18 A313 A312 A311 | A10 A277 A276 A275 A99 A16 A97 A96 | A17 A82 A81 A80 A79 A78 A77 A76 A75 A74 A73 A72 A71 A70 A69 A68 A67 A66 A65 A64 A63 A62 A61 A60 A59 A58 A57 A56 A55 A54 A53 A52 A23 A10 | A10 A23 L3 A17 | A18 A11 A17 A82 A83 | A18 A228 A227 A226 A225 A224 A17 A11 | A23 L29 A24 A10 | A10 A24 A147 A23 | A201 A202 A203 A204 A113 A112 A111 A110 A109 A108 A17 A10 | A10 A17 A182 A183 A184 A185 A186 A187 A188 A189 A190 A191 A192 A193 A194 A195 A196 A197 A198 A199 A200 A201 | A116 A117 A118 A119 A120 A121 A122 A123 A124 A125 A126 A127 A128 A129 A130 A131 A132 A133 A134 A135 A136 A137 A138 A139 A140 A141 A142 A143 A144 A145 A146 A147 A23 A50 A51 A52 A53 A54 A55 A56 A57 A58 A59 A60 A61 A62 A63 A64 A65 A66 A67 A68 A69 A70 A71 A72 A73 A74 A75 A76 A77 A78 A79 A80 A81 A82 A17 A11 A6 | A11 A6 A215 A214 A213 A212 A211 A210 A209 A208 A207 A206 A205 A204 A113 A114 A115 A116 | A17 A182 A181 A180 | A16 A108 A107 A105 A18 A317 A316 A315 A10 | A10 A17 A108 A16 | A311 A312 A313 A18 | A18 A313 A314 A315 A10 A317 A318 A277 A278 A279 A280 A281 A282 A283 A284 A285 A286 A287 A288 A289 A290 A291 A292 A293 A294 A295 A296 A297 A298 A299 A300 A301 A302 A303 A304 A305 A306 A307 A308 A309 A310 A311 | A10 A318 A319 A103 A320 A273 A274 A275 A100 A99 A276 A277 | A96 A97 A16 | A16 A97 A98 A99 A18 A225 A226 A228 A229 A230 A231 A232 A89 A90 A91 A233 A92 A93 A94 A95 A96 | A89 A234 A235 | A17 A224 A223 A222 A221 A220 A6 A11 | A18 A226 A227 A228 | A24 L29 L23 L24 L3 L11 L7 L13 L12 A3 A28 L20 A10 | A10 A24 A49 A48 A47 A46 A45 A44 A43 A42 A41 A40 A39 A38 A37 A36 A35 A34 A33 A32 A31 A150 A149 A148 A147 | A147 A24 A49 A50 A23 | A18 A315 A10 | A10 A315 A314 A313 A18 | A108 A17 A224 A225 A18 A16 A105 A106 A107 | A16 A107 A108 | A318 A317 A10 | A10 A317 A18 A105 A104 A103 A319 A318 | A16 A99 A98 A97 | A234 A233 A91 A232 A89 | A23 A52 A51 A50 A49 A24 A10 | A10 A24 L3 A23 | A17 A108 A109 A110 A111 A112 A113 A204 A205 A206 A207 A208 A209 A210 A211 A212 A213 A214 A215 A6 A216 A217 A218 A220 A221 A222 A223 A224 | A226 A225 A18 | A147 A148 A149 A150 A31 A32 A33 A34 A35 A36 A37 A38 A39 A40 A41 A42 A43 A44 A45 A46 A47 A48 A49 A24 | A23 A51 A50 | L1 L2 A23 L24 L21 L30 | A315 A18 A317 A10 | A315 A316 A317 A18 | A107 A106 A105 A16 | A99 A275 A100 A101 A102 A103 A320 A319 A104 A105 A18 A16 | A232 A91 A90 A89 | A23 A51 A52 | A6 A218 A217 A216 | A16 A18 A105 | A319 A320 A103 | A99 A100 A275 | A91 A233 A232 | L20 A28 L3 | A23 L3 L16 L15 L14 | L14 A24 L3 A23 | L2 L3 A23 | A23 L3 A24 L24 | A103 A102 A101 A100 A275 A274 A273 A320 | L14 L3 A24 | L3 L12 A3 L13 L7 L11 | L12 A3 | A3 L12 | A19 | A20 | A26 L18 A25 L17 picked at (24.833671, -4.407291)
extrude "Extrusion2" add sketch "Sketch1" against normal blind 3.1 contours A2 A11 A10 A18 L3 L0 | A2 A253 A252 A251 A250 A249 A248 A247 A246 A245 A244 A243 A242 A241 A240 A239 A238 A237 A236 A10 A11 | A11 A18 A178 A177 A176 A175 A174 A173 A172 A171 A170 A169 A168 A167 A166 A165 A164 A163 A162 A161 A160 A159 A158 A157 A156 A155 A154 A153 A152 A2 | A2 A152 A153 A154 A155 A156 A157 A158 A159 A160 A161 A162 A163 A164 A165 A166 A167 A168 A169 A170 A171 A172 A173 A174 A175 A176 A177 A178 A18 A16 A10 A236 A237 A238 A239 A240 A241 A242 A243 A244 A245 A246 A247 A248 A249 A250 A251 A252 A253 | A18 L0 A17 A11 | A11 A17 A178 A18 | A11 A88 A87 A86 A85 A84 A83 A18 A10 | A10 A236 A235 A89 A88 A11 | A17 L1 L29 A23 A10 A11 | A11 A10 A201 A200 A199 A198 A197 A196 A195 A194 A193 A192 A191 A190 A189 A188 A187 A186 A185 A184 A183 A182 A17 A180 A179 A178 | A178 A17 A180 A181 A182 A10 A16 A18 | A10 A16 A96 A95 A94 A93 A92 A91 A233 A234 A89 A235 A236 | A18 A83 A82 A17 A10 | A10 A17 L3 A18 | A88 A89 A235 A234 A232 A231 A230 A229 A228 A18 A11 | A11 A18 A83 A84 A85 A86 A87 A88 | A11 A116 A115 A114 A113 A204 A203 A202 A201 A10 | A10 A23 A147 A146 A145 A144 A143 A142 A141 A140 A139 A138 A137 A136 A135 A134 A133 A132 A131 A130 A129 A128 A127 A126 A125 A124 A123 A122 A121 A120 A119 A118 A117 A116 A11 | A178 A179 A180 A17 | A17 L0 L1 | A17 A82 A81 A80 A79 A78 A77 A76 A75 A74 A73 A72 A71 A70 A69 A68 A67 A66 A65 A64 A63 A62 A61 A60 A59 A58 A57 A56 A55 A54 A53 A52 A23 A10 | A10 A23 L3 A17 | A18 A11 A17 A82 A83 | A18 A228 A227 A226 A225 A224 A17 A11 | A23 L29 A24 A10 | A10 A24 A147 A23 | A201 A202 A203 A204 A113 A112 A111 A110 A109 A108 A17 A10 | A10 A17 A182 A183 A184 A185 A186 A187 A188 A189 A190 A191 A192 A193 A194 A195 A196 A197 A198 A199 A200 A201 | A116 A117 A118 A119 A120 A121 A122 A123 A124 A125 A126 A127 A128 A129 A130 A131 A132 A133 A134 A135 A136 A137 A138 A139 A140 A141 A142 A143 A144 A145 A146 A147 A23 A50 A51 A52 A53 A54 A55 A56 A57 A58 A59 A60 A61 A62 A63 A64 A65 A66 A67 A68 A69 A70 A71 A72 A73 A74 A75 A76 A77 A78 A79 A80 A81 A82 A17 A11 A6 | A11 A6 A215 A214 A213 A212 A211 A210 A209 A208 A207 A206 A205 A204 A113 A114 A115 A116 | A17 A182 A181 A180 | A10 A17 A108 A16 | A16 A97 A98 A99 A18 A225 A226 A228 A229 A230 A231 A232 A89 A90 A91 A233 A92 A93 A94 A95 A96 | A89 A234 A235 | A17 A224 A223 A222 A221 A220 A6 A11 | A18 A226 A227 A228 | A24 L29 L23 L24 L3 L11 L7 L13 L12 A3 A28 L20 A10 | A10 A24 A49 A48 A47 A46 A45 A44 A43 A42 A41 A40 A39 A38 A37 A36 A35 A34 A33 A32 A31 A150 A149 A148 A147 | A147 A24 A49 A50 A23 | A108 A17 A224 A225 A18 A16 A105 A106 A107 | A16 A99 A98 A97 | A234 A233 A91 A232 A89 | A23 A52 A51 A50 A49 A24 A10 | A10 A24 L3 A23 | A17 A108 A109 A110 A111 A112 A113 A204 A205 A206 A207 A208 A209 A210 A211 A212 A213 A214 A215 A6 A216 A217 A218 A220 A221 A222 A223 A224 | A226 A225 A18 | A147 A148 A149 A150 A31 A32 A33 A34 A35 A36 A37 A38 A39 A40 A41 A42 A43 A44 A45 A46 A47 A48 A49 A24 | A23 A51 A50 | L1 L2 A23 L24 L21 L30 | A107 A106 A105 A16 | A232 A91 A90 A89 | A23 A51 A52 | A6 A218 A217 A216 | A91 A233 A232 | L20 A28 L3 | A23 L3 L16 L15 L14 | L14 A24 L3 A23 | L2 L3 A23 | A23 L3 A24 L24 | L14 L3 A24 | L3 L12 A3 L13 L7 L11 | L12 A3 | A3 L12 | A19 | A20 | A26 L18 A25 L17 picked at (24.833671, -4.407291)
extrude "Extrusion3" add sketch "Sketch1" against normal blind 6.2 contours A2 A11 A10 A18 L3 L0 | A2 A253 A252 A251 A250 A249 A248 A247 A246 A245 A244 A243 A242 A241 A240 A239 A238 A237 A236 A10 A11 | A11 A18 A178 A177 A176 A175 A174 A173 A172 A171 A170 A169 A168 A167 A166 A165 A164 A163 A162 A161 A160 A159 A158 A157 A156 A155 A154 A153 A152 A2 | A2 A152 A153 A154 A155 A156 A157 A158 A159 A160 A161 A162 A163 A164 A165 A166 A167 A168 A169 A170 A171 A172 A173 A174 A175 A176 A177 A178 A18 A16 A10 A236 A237 A238 A239 A240 A241 A242 A243 A244 A245 A246 A247 A248 A249 A250 A251 A252 A253 | A18 L0 A17 A11 | A11 A17 A178 A18 | A17 L1 L29 A23 A10 A11 | A11 A10 A201 A200 A199 A198 A197 A196 A195 A194 A193 A192 A191 A190 A189 A188 A187 A186 A185 A184 A183 A182 A17 A180 A179 A178 | A178 A17 A180 A181 A182 A10 A16 A18 | A10 A17 L3 A18 | A178 A179 A180 A17 | A17 L0 L1 | A10 A23 L3 A17 | A23 L29 A24 A10 | A10 A17 A182 A183 A184 A185 A186 A187 A188 A189 A190 A191 A192 A193 A194 A195 A196 A197 A198 A199 A200 A201 | A17 A182 A181 A180 | A24 L29 L23 L24 L3 L11 L7 L13 L12 A3 A28 L20 A10 | A10 A24 L3 A23 | L1 L2 A23 L24 L21 L30 | L20 A28 L3 | A23 L3 L16 L15 L14 | L14 A24 L3 A23 | L2 L3 A23 | A23 L3 A24 L24 | L14 L3 A24 | L3 L12 A3 L13 L7 L11 | L12 A3 | A3 L12 | A19 | A20 | A26 L18 A25 L17 picked at (24.833671, -4.407291)
ref_plane "Work Plane1" through (6.581406, -41.040807, -9.3) normal (0, 0, -1) x (0.0707652, 0.997493, 0)
extrude "Extrusion4" add sketch "Sketch1" against normal up to surface (9.3 mm away) contours A2 A11 A10 A18 L3 L0 | A18 L0 A17 A11 | A17 L1 L29 A23 A10 A11 | A10 A17 L3 A18 | A17 L0 L1 | A10 A23 L3 A17 | A23 L29 A24 A10 | A24 L29 L23 L24 L3 L11 L7 L13 L12 A3 A28 L20 A10 | A10 A24 L3 A23 | L1 L2 A23 L24 L21 L30 | L20 A28 L3 | A23 L3 L16 L15 L14 | L14 A24 L3 A23 | L2 L3 A23 | A23 L3 A24 L24 | L14 L3 A24 | L3 L12 A3 L13 L7 L11 | L12 A3 | A3 L12 | A19 | A20 | A26 L18 A25 L17 picked at (24.833671, -4.407291)
sketch "Sketch2" plane through (0, 0, 0) normal (0, 0, 1) x (1, 0, 0)
  line L0 (23.1, 0) -> (0, 0)
  line L1 (0, 0) -> (0, -29.4)
  line L2 (0, -29.4) -> (23.1, -29.4)
  line L3 (23.1, -29.4) -> (23.1, 0)
  arc A0 (24.939129, -23.498315) -> (27.439129, -19.168188) centre (14.7, -14.7) ccw
  line L4 (27.439129, -19.168188) -> (23.43749, -16.857841)
  arc A1 (20.93749, -21.187968) -> (23.43749, -16.857841) centre (14.7, -14.7) ccw construction
  line L5 (20.93749, -21.187968) -> (24.939129, -23.498315)
  line L6 (5.96251, -12.542159) -> (1.960875, -10.231814)
  arc A2 (4.460875, -5.901687) -> (1.960875, -10.231814) centre (14.7, -14.7) ccw
  line L7 (4.460875, -5.901687) -> (8.46251, -8.212032)
  line L8 (24.939129, -23.498315) -> (23.1, -23.498315)
  line L9 (20.93749, -21.187968) -> (23.43749, -16.857841)
  line L10 (20.93749, -21.187968) -> (23.1, -21.187968)
  line L11 (8.46251, -8.212032) -> (23.1, -8.212032)
  line L12 (5.96251, -12.542159) -> (8.46251, -8.212032)
  line L13 (4.460875, -5.901687) -> (23.1, -5.901687)
  line L14 (6.887728, -8.457532) -> (4.702907, -7.196125)
  arc A3 (4.702907, -7.196125) -> (3.202907, -9.794201) centre (14.7, -14.7) ccw
  line L15 (3.202907, -9.794201) -> (5.387728, -11.055608)
  arc A4 (6.887728, -8.457532) -> (5.387728, -11.055608) centre (14.7, -14.7) ccw
  arc A5 (24.697093, -22.203875) -> (26.197093, -19.605799) centre (14.7, -14.7) ccw
  line L16 (26.197093, -19.605799) -> (24.012272, -18.344392)
  arc A6 (22.512272, -20.942468) -> (24.012272, -18.344392) centre (14.7, -14.7) ccw
  line L17 (22.512272, -20.942468) -> (24.697093, -22.203875)
  circle A7 centre (14.7, -14.7) radius 5
  circle A8 centre (14.7, -14.7) radius 14
  circle A9 centre (14.7, -14.7) radius 14.7
  circle A10 centre (14.7, -14.7) radius 14
  circle A11 centre (14.7, -14.7) radius 5
  arc A12 (8.46251, -8.212032) -> (5.96251, -12.542159) centre (14.7, -14.7) ccw construction
  line L18 (23.1, -23.498315) -> (27.4, -23.498315)
  line L19 (27.4, -23.498315) -> (27.4, -21.187968)
  line L20 (27.4, -21.187968) -> (23.1, -21.187968)
  line L21 (23.1, -5.901687) -> (27.4, -5.901687)
  line L22 (27.4, -6.5) -> (27.4, 0)
  line L23 (23.1, -8.212032) -> (27.4, -8.212032)
  line L24 (27.4, -8.212032) -> (27.4, -5.901687)
  line L25 (2.5, -1) -> (2.5, -17.5)
  line L26 (3, -7.965017) -> (3, -10.831753)
  point P0 (0, 0)
  point P1 (23.1, -26.519052)
  point P2 (23.1, -18.857359)
  point P3 (6.039746, -9.7)
  point P4 (23.1, -20.043559)
  point P5 (23.1, -26.519057)
  point P6 (23.1, -22.436494)
  point P7 (23.1, -17.44239)
  dimension "d34" = 6.3
  dimension "d35" = 1
  dimension "d36" = 1
  dimension "d39" = 1
  dimension "d41" = 1
  dimension "d50" = 1
  dimension "d51" = 1
  dimension "d53" = 1
  dimension "d55" = 1
  dimension "d157" = 2
  dimension "d205" = 0.5
  constraints: 42 end point, 10 point on circle, 7 perpendicular, 7 point on line, 5 centre point, 5 coincident, 5 parallel, 4 tangent, 3 horizontal, 1 collinear
  measures "d34" distance edge to line of A9 L3
  measures "d35" distance between parallel lines of L4 L16
  measures "d36" distance between parallel lines of L5 L17
  measures "d39" distance between parallel lines of L7 L14
  measures "d41" distance between parallel lines of L6 L15
  measures "d50" radial gap between concentric circles of A1 A6
  measures "d51" radial gap between concentric circles of A5 A0
  measures "d53" radial gap between concentric circles of A3 A2
  measures "d55" radial gap between concentric circles of A4 A12
  measures "d157" distance edge to line of A9 L19
  measures "d205" distance between parallel lines of L26 L25
extrude "Extrusion5" cut sketch "Sketch2" against normal blind 4 contours L21 L22 L24 A9 | A9 L24 L23 A8 L21 | L21 A8 L23 L3 | L3 L11 L7 L13 | L7 L12 L6 L26 A2 | L3 A6 L17 L10 L9 | L5 L10 L17 L3 | L3 L10 L17 A6 | L17 L10 L3 | A4 L15 A3 L14 | A7
sketch "Sketch3" plane through (27.4, 0, -9.3) normal (0, 0, -1) x (-1, 0, 0)
  circle A0 centre (18.356854, -61.293926) radius 1.05643
  circle A1 centre (7.043146, -49.980218) radius 1.05643
  circle A2 centre (12.7, -55.637072) radius 14.7
  circle A3 centre (12.7, -14.7) radius 14.7
  line L0 (4.3, -65.837072) -> (27.4, -65.837072)
  line L1 (27.4, -65.837072) -> (27.4, 0)
  line L2 (27.4, 0) -> (4.3, 0)
  line L3 (0, -6.5) -> (0, 0)
  line L4 (0, -6.5) -> (0, 0)
  line L5 (0, 0) -> (27.4, 0)
  line L6 (4.3, 0) -> (0, 0)
  line L7 (25.9, -1) -> (25.9, -17)
  line L8 (24.9, -1) -> (25.9, -1)
  line L9 (24.9, -17) -> (24.9, -1)
  line L10 (24.9, -17) -> (25.9, -17)
  line L11 (27.4, -19.5) -> (4.3, -19.5)
  line L12 (4.3, -19.5) -> (0, -19.5)
  line L13 (0, -19.5) -> (0, -6.5) construction
  line L14 (0, -19.5) -> (0, -13.5)
  line L15 (0, -13.5) -> (24.9, -13.5)
  line L16 (24.9, -13.5) -> (24.9, -17.5)
  line L17 (24.9, -17.5) -> (26.4, -17.5)
  line L18 (26.4, -17.5) -> (26.4, -15)
  line L19 (26.4, -15) -> (27.4, -15)
  line L20 (27.4, -3.5) -> (26.4, -3.5)
  line L21 (26.4, -3.5) -> (26.4, -1)
  line L22 (26.4, -1) -> (24.9, -1)
  line L23 (24.9, -1) -> (24.9, -6.5)
  line L24 (4.3, -6.5) -> (0, -6.5)
  line L25 (24.9, -6.5) -> (0, -6.5)
  circle A4 centre (7.043146, -49.980218) radius 2.25
  circle A5 centre (18.356854, -61.293926) radius 2.25
  line L26 (25.9, -1) -> (25.9, -17)
  line L27 (24.9, -1) -> (25.9, -1)
  line L28 (24.9, -17) -> (24.9, -1)
  line L29 (24.9, -17) -> (25.9, -17)
  circle A6 centre (12.7, -14.7) radius 14.7
  circle A7 centre (12.7, -14.7) radius 14
  circle A8 centre (12.7, -55.637072) radius 14.7
  circle A9 centre (12.7, -55.637072) radius 14
  circle A10 centre (18.356854, -61.293926) radius 1.05643
  circle A11 centre (7.043146, -49.980218) radius 1.05643
  circle A12 centre (12.7, -55.637072) radius 5
  circle A13 centre (12.7, -55.637072) radius 14
  point P0 (24.9, -1)
  point P1 (25.9, -1)
  dimension "d81" = 4.5
  dimension "d83" = 2.5
  dimension "d84" = 6
  dimension "d85" = 0.5
  dimension "d86" = 2.5
  dimension "d87" = 0.5
  dimension "d88" = 0
  dimension "d89" = 2.5
  dimension "d90" = 0.5
  dimension "d91" = 0
  dimension "d92" = 0
  dimension "d95" = 4.5
  dimension "d96" = 4.5
  constraints: 46 end point, 8 perpendicular, 6 centre point, 6 coincident, 5 point on line, 5 tangent, 4 horizontal, 3 vertical, 1 collinear, 1 parallel
  measures "d81" distance edge to line of A2 L0
  measures "d83" distance between parallel lines of L11 L10
  measures "d84" distance between parallel lines of L11 L15
  measures "d85" distance between parallel lines of L18 L7
  measures "d86" distance between parallel lines of L17 L19
  measures "d87" distance between parallel lines of L17 L10
  measures "d88" distance between parallel lines of L9 L16
  measures "d89" distance between parallel lines of L22 L20
  measures "d90" distance between parallel lines of L7 L21
  measures "d91" distance between parallel lines of L22 L8
  measures "d92" distance between parallel lines of L9 L23
  measures "d95" diameter of A4
  measures "d96" diameter of A5
ref_plane "Work Plane3" through (1, -19, -16) normal (0, 0, 1) x (1, 0, 0)